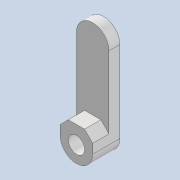
# Autodesk Inventor part: stand_1
Saved by Autodesk Inventor 2020 (Build 240168000, 168)
## iProperties
Created: 2021-07-20
Part Number: stand_1
Material: Generic
Document SubType Name: Modeling
Designer: Shuang Peng
Density: 1 g/cm^3
Appearance: Default
Author: Shuang Peng
Autodesk Inventor part; units mm, degrees
ref_plane "YZ Plane" through (0, 0, 0) normal (1, 0, 0) x (0, 1, 0)
ref_plane "XZ Plane" through (0, 0, 0) normal (0, 1, 0) x (-1, 0, 0)
ref_plane "XY Plane" through (0, 0, 0) normal (0, 0, 1) x (1, 0, 0)
sketch "Sketch1" plane through (0, 0, 0) normal (0, 0, 1) x (1, 0, 0)
  circle A0 centre (0, 0) radius 3
  line L0 (0, 0) -> (0, 30) construction
  line L1 (6, 0) -> (6, 30)
  line L2 (-6, 30) -> (-6, 0)
  arc A1 (-6, 0) -> (6, 0) centre (0, 0) ccw
  arc A2 (6, 30) -> (-6, 30) centre (0, 30) ccw
  point P0 (0, 15)
  dimension "d0" = 6
  dimension "d1" = 30
  dimension "d2" = 12
  constraints: 8 end point, 4 point on circle, 4 tangent, 3 centre point, 1 coincident, 1 midpoint, 1 parallel, 1 vertical
  measures "d0" diameter of A0
  measures "d1" distance of L0.start L0.end
  measures "d2" diameter of A2
extrude "Extrusion1" add sketch "Sketch1" along normal blind 10
sketch "Sketch2" plane through (0, 0, 10) normal (0, 0, 1) x (1, 0, 0)
  line L0 (-6, 30) -> (-6, 0) projected
  arc A0 (-6, 0) -> (6, 0) centre (0, 0) ccw projected
  line L1 (6, 0) -> (6, 30) projected
  arc A1 (6, 30) -> (-6, 30) centre (0, 30) ccw projected
  circle A2 centre (0, 0) radius 3 projected
  line L2 (13.5, 6.5) -> (13.5, -6.5)
  line L3 (13.5, -6.5) -> (-13.5, -6.5)
  line L4 (-13.5, -6.5) -> (-13.5, 6.5)
  line L5 (-13.5, 6.5) -> (13.5, 6.5)
  line L6 (13.5, 6.5) -> (-13.5, -6.5) construction
  line L7 (13.5, -6.5) -> (-13.5, 6.5) construction
  point P0 (-6, 6.5)
  point P1 (6, 6.5)
  dimension "d5" = 13
  dimension "d6" = 27
  constraints: 12 end point, 2 midpoint, 2 parallel, 1 perpendicular, 1 vertical
  measures "d5" distance of L2.start L2.end
  measures "d6" distance of L2.end L3.end
extrude "Extrusion2" cut sketch "Sketch2" against normal blind 6 contours A1 L1 L5 L0
chamfer "Chamfer1" distance 3 angle 45 2 edges at (-6, 6.5, 7) (6, 6.5, 7)
sketch "Sketch3" plane through (0, 0, 0) normal (0, 0, -1) x (-1, 0, 0)
  line L0 (6, 30) -> (6, 0) projected
  arc A0 (6, 30) -> (-6, 30) centre (0, 30) ccw projected
  line L1 (-6, 0) -> (-6, 30) projected
  arc A1 (-6, 0) -> (6, 0) centre (0, 0) ccw projected
  circle A2 centre (0, 0) radius 3 projected
  line L2 (6, 30) -> (6, 0) projected
  line L3 (-6, 30) -> (6, 30)
  constraints: 2 end point, 1 horizontal
extrude "Extrusion3" cut sketch "Sketch3" against normal blind 6 contours L3 A0
sketch "Sketch4" plane through (0, 0, 4) normal (0, 0, 1) x (1, 0, 0)
  line L0 (6, 30) -> (-6, 30) projected
  line L1 (-6, 3.5) -> (-6, 30) projected
  line L2 (-3, 6.5) -> (-6, 3.5) projected
  line L3 (3, 6.5) -> (-3, 6.5) projected
  line L4 (6, 3.5) -> (3, 6.5) projected
  line L5 (6, 30) -> (6, 3.5) projected
  arc A0 (-23.6294, 8.164) -> (-15.9746, 19.2305) centre (0, 0) ccw projected
  line L6 (6, 30) -> (6, 3.5) projected
  line L7 (6, 30) -> (18.1372, 17.2059)
  line L8 (-6, 30) -> (-18.1372, 17.2059)
  line L9 (4.0098, 35.0039) -> (10.8922, 27.749)
  line L10 (10.8922, 27.749) -> (7.9902, 24.9961)
  line L11 (7.9902, 24.9961) -> (1.1078, 32.251)
  line L12 (1.1078, 32.251) -> (4.0098, 35.0039)
  line L13 (6, 30) -> (-6, 30) projected
  line L14 (4.0098, 35.0039) -> (7.9902, 24.9961) construction
  line L15 (10.8922, 27.749) -> (1.1078, 32.251) construction
  line L16 (-1.1078, 32.251) -> (-7.9902, 24.9961)
  line L17 (-7.9902, 24.9961) -> (-10.8922, 27.749)
  line L18 (-10.8922, 27.749) -> (-4.0098, 35.0039)
  line L19 (-4.0098, 35.0039) -> (-1.1078, 32.251)
  line L20 (-1.1078, 32.251) -> (-10.8922, 27.749) construction
  line L21 (-7.9902, 24.9961) -> (-4.0098, 35.0039) construction
  line L22 (1.1078, 32.251) -> (-1.1078, 32.251)
  line L23 (6, 30) -> (2.5588, 33.6274)
  line L24 (-6, 30) -> (-2.5588, 33.6274)
  line L25 (7.9902, 24.9961) -> (-7.9902, 24.9961)
  point P0 (6, 24.9961)
  point P1 (9.4412, 26.3726)
  point P2 (-9.4412, 26.3726)
  point P3 (-6, 24.9961)
  point P4 (-6, 27.094)
  point P5 (-3.2432, 30)
  point P6 (3.2432, 30)
  point P7 (6, 27.094)
  dimension "d14" = 10
  dimension "d15" = 4
  dimension "d16" = 10
  dimension "d17" = 4
  constraints: 36 end point, 6 midpoint, 6 parallel, 3 perpendicular, 2 point on circle, 2 tangent
  measures "d14" distance of L9.start L9.end
  measures "d15" distance of L9.end L10.end
  measures "d16" distance of L16.start L16.end
  measures "d17" distance of L16.end L17.end
extrude "Extrusion4" add sketch "Sketch4" against normal blind 15 contours L5 L11 L0 | L7 L10 L11 L5 | L0 L11 L12 L23 | L0 L16 L22 L11 | L11 L25 L5 | L16 L1 L0 | L0 L24 L19 L16 | L1 L16 L17 L8 | L1 L25 L16
sketch "Sketch5" plane through (0, 0, -11) normal (0, 0, -1) x (-1, 0, 0)
  line L0 (1.1078, 32.251) -> (-1.1078, 32.251) projected
  line L1 (-1.1078, 32.251) -> (-2.5588, 33.6274) projected
  line L2 (-2.5588, 33.6274) -> (-9.4412, 26.3726) projected
  line L3 (-9.4412, 26.3726) -> (-7.9902, 24.9961) projected
  line L4 (-7.9902, 24.9961) -> (-6, 24.9961) projected
  line L5 (-6, 24.9961) -> (-6, 27.094) projected
  line L6 (-6, 27.094) -> (-3.2432, 30) projected
  line L7 (-3.2432, 30) -> (3.2432, 30) projected
  line L8 (3.2432, 30) -> (6, 27.094) projected
  line L9 (6, 27.094) -> (6, 24.9961) projected
  line L10 (6, 24.9961) -> (7.9902, 24.9961) projected
  line L11 (7.9902, 24.9961) -> (9.4412, 26.3726) projected
  line L12 (9.4412, 26.3726) -> (2.5588, 33.6274) projected
  line L13 (2.5588, 33.6274) -> (1.1078, 32.251) projected
  line L14 (-7.9902, 24.9961) -> (-6, 27.094)
  line L15 (7.9902, 24.9961) -> (6, 27.094)
  point P0 (0, 0)
  constraints: 4 end point
extrude "Extrusion5" cut sketch "Sketch5" against normal up to surface (11 mm away) contours L10 L9 L15 | L14 L5 L4
thicken "Thicken1" operation add thickness 1 both sides no extend neighbours yes toward (0.6882359, 0.7254869, 0) faces at (-8.9575, 25.9137, -2.3333)
thicken "Thicken2" operation add thickness 1 both sides no extend neighbours yes toward (-0.6882359, 0.7254869, 0) faces at (8.9575, 25.9137, -2.3333)
sketch "Sketch6" plane through (-1.1078, 32.251, 4) normal (0.6882359, 0.7254869, 0) x (0.7254869, -0.6882359, 0)
  line L0 (-2, 12.5) -> (-3.1464, 13.6464)
  line L1 (-3.1464, 11.3536) -> (-2, 12.5)
  line L2 (-2, 0) -> (-2, 15) projected
  circle A0 centre (-2, 12.5) radius 1.25
  point P0 (23, 4)
  point P1 (-2, 13.75)
  point P2 (-2, 11.25)
  dimension "d27" = 2.5
  constraints: 4 end point, 1 centre point, 1 coincident, 5 other
  measures "d27" diameter of A0
extrude "Extrusion6" cut sketch "Sketch6" against normal blind 15 contours L2 A0
sketch "Sketch7" plane through (-1.1078, 32.251, 4) normal (0.6882359, 0.7254869, 0) x (0.7254869, -0.6882359, 0)
  line L0 (-2, 8.5) -> (-3.1464, 7.3536)
  line L1 (-3.1464, 9.6464) -> (-2, 8.5)
  line L2 (-2, 0) -> (-2, 11.25) projected
  circle A0 centre (-2, 8.5) radius 1.25
  point P0 (23, 4)
  point P1 (-2, 9.75)
  point P2 (-2, 7.25)
  dimension "d30" = 2.5
  constraints: 4 end point, 1 centre point, 1 coincident, 5 other
  measures "d30" diameter of A0
extrude "Extrusion7" cut sketch "Sketch7" against normal blind 15 contours L2 A0
chamfer "Chamfer2" distance 2 angle 45 2 edges at (-5.6559, 30.3627, 4) (5.6559, 30.3627, 4)
sketch "Sketch8" plane through (0, 0, -11) normal (0, 0, -1) x (-1, 0, 0)
  arc A0 (23.3037, 11.8564) -> (25.9335, 3.3299) centre (0, 0) ccw projected
  circle A1 centre (0, 0) radius 3 projected
  line L0 (7.302, 25.7216) -> (3.2432, 30) projected
  line L1 (3.2432, 30) -> (-3.2432, 30) projected
  line L2 (-3.2432, 30) -> (-7.302, 25.7216) projected
  line L3 (-7.302, 25.7216) -> (-6.5372, 24.9961) projected
  line L4 (-6, 24.9961) -> (-6.5372, 24.9961) projected
  line L5 (-6, 0) -> (-6, 24.9961) projected
  arc A2 (-6, 0) -> (6, 0) centre (0, 0) ccw projected
  line L6 (6, 24.9961) -> (6, 0) projected
  line L7 (6.5372, 24.9961) -> (6, 24.9961) projected
  line L8 (6.5372, 24.9961) -> (7.302, 25.7216) projected
  line L9 (-5.2726, 27.8608) -> (5.2726, 27.8608)
  constraints: 2 end point, 2 midpoint
extrude "Extrusion8" add sketch "Sketch8" against normal up to surface (11 mm away) contours L9 L2 L1 L0
ref_plane "Work Plane2" through (0, 36.3248, -3.25) normal (-1, 0, 0) x (0, 0, 1)
mirror "Mirror2" about plane through (0, 36.3248, -3.25) normal (-1, 0, 0) of "Extrusion7", "Extrusion6"
thicken "Thicken3" operation add thickness 1 both sides no extend neighbours yes toward (0, 1, 0) faces at (1.7575, 27.8608, -7.3333)
thicken "Thicken4" operation add thickness 2 both sides no extend neighbours yes toward (0, 0, -1) faces at (0.3693, 29.9908, -11)
fillet "Fillet2" radius 3 2 edges at (-6, 24.9961, 2) (6, 24.9961, 2)
fillet "Fillet3" radius 3 3 edges at (-5.813, 27.2912, 0) (0, 28.8608, 0) (5.813, 27.2912, 0)
sketch "Sketch9" plane through (-2.5588, 33.6274, -13) normal (-0.7254869, 0.6882359, 0) x (0, 0, 1)
  line L0 (3.25, -9) -> (3.25, 0) projected
  line L1 (3.25, 0) -> (0, 0) projected
  line L2 (0, -9) -> (0, 0) projected
  line L3 (3.25, -9) -> (0, -9) projected
  line L4 (15, 0) -> (15, -9) projected
  line L5 (15, 0) -> (9.75, 0) projected
  line L6 (9.75, 0) -> (9.75, -9) projected
  line L7 (15, -9) -> (9.75, -9) projected
  line L8 (3.25, -9) -> (3.25, 0) projected
  line L9 (17, 0) -> (0, 0) projected
  line L10 (3.25, 0) -> (0, 0)
  line L11 (1.625, 0) -> (1.625, -9)
  line L12 (10, -9) -> (0, -9) projected
  line L13 (1.625, -3) -> (1.625, -6) construction
  line L14 (1.275, -3) -> (1.275, -6)
  line L15 (1.975, -6) -> (1.975, -3)
  arc A0 (1.975, -3) -> (1.275, -3) centre (1.625, -3) ccw
  arc A1 (1.275, -6) -> (1.975, -6) centre (1.625, -6) ccw
  line L16 (1.625, -4.5) -> (11.125, -4.5)
  line L17 (11.125, -3) -> (11.125, -6) construction
  line L18 (10.775, -3) -> (10.775, -6)
  line L19 (11.475, -6) -> (11.475, -3)
  arc A2 (11.475, -3) -> (10.775, -3) centre (11.125, -3) ccw
  arc A3 (10.775, -6) -> (11.475, -6) centre (11.125, -6) ccw
  point P0 (13, -22.6352)
  dimension "d44" = 1.5
  dimension "d45" = 0.7
  dimension "d46" = 9.5
  dimension "d47" = 1.5
  dimension "d48" = 0.7
  constraints: 22 end point, 8 point on circle, 8 tangent, 4 centre point, 4 midpoint, 2 parallel, 2 perpendicular, 2 point on line, 1 horizontal, 1 vertical
  measures "d44" distance of L16.start L13.end
  measures "d45" diameter of A1
  measures "d46" distance of L16.start L16.end
  measures "d47" distance of L16.end L17.end
  measures "d48" diameter of A3
extrude "Extrusion9" cut sketch "Sketch9" against normal blind 15 contours L16 L11 A0 L15 | L15 A1 L11 L16 | A1 L14 A0 L11 | A2 L19 A3 L18
mirror "Mirror3" about plane through (0, 36.3248, -3.25) normal (-1, 0, 0) of "Extrusion9"
fillet "Fillet4" radius 2 8 edges at (4.3239, 28.8608, -12.3625) (4.313, 28.8352, -2.6092) (4.3239, 28.8608, -7.0125) (3.6847, 27.3732, -0.4092) (-3.6847, 27.3732, -0.4092) (-4.313, 28.8352, -2.6092) (-4.3239, 28.8608, -7.0125) (-4.3239, 28.8608, -12.3625)
ref_plane "Work Plane3" through (0, 0, 8) normal (0, 0, 1) x (1, 0, 0)
sketch "Sketch10" plane through (0, 0, 8) normal (0, 0, 1) x (1, 0, 0)
  circle A0 centre (0, 0) radius 3 projected
  circle A1 centre (0, 0) radius 2
  dimension "d53" = 1
  constraints: 1 centre point, 1 coincident
  measures "d53" radial gap between concentric circles of A0 A1
extrude "Extrusion10" add sketch "Sketch10" against normal blind 6
chamfer "Chamfer3" distance 1 angle 45 2 edges at (-2, 0, 8) (-2, 0, 2)
thicken "Thicken5" operation add thickness 1 both sides no extend neighbours yes toward (0, -1, 0) faces at (-1, 6.5, 8)
sketch "Sketch11" plane through (0, 0, 4) normal (0, 0, 1) x (1, 0, 0)
  line L0 (1.1078, 32.251) -> (7.302, 25.7216) projected
  line L1 (1.1078, 32.251) -> (-1.1078, 32.251) projected
  line L2 (-7.302, 25.7216) -> (-1.1078, 32.251) projected
  line L3 (-7.302, 25.7216) -> (-6.5372, 24.9961) projected
  arc A0 (-6, 23.283) -> (-6.5372, 24.9961) centre (-9, 23.283) ccw projected
  line L4 (-6, 3.5) -> (-6, 23.283) projected
  line L5 (-4, 5.5) -> (-6, 3.5) projected
  line L6 (4, 5.5) -> (-4, 5.5) projected
  line L7 (6, 3.5) -> (4, 5.5) projected
  line L8 (6, 23.283) -> (6, 3.5) projected
  arc A1 (6.5372, 24.9961) -> (6, 23.283) centre (9, 23.283) ccw projected
  line L9 (6.5372, 24.9961) -> (7.302, 25.7216) projected
  line L10 (0, 32.251) -> (0, 27.251)
  line L11 (0, 27.251) -> (0, 21.251)
  line L12 (0, 21.251) -> (0, 9.251)
  circle A2 centre (0, 27.251) radius 1.5
  circle A3 centre (0, 21.251) radius 1.5
  circle A4 centre (0, 9.251) radius 1.5
  line L13 (0, 15.251) -> (3, 15.251)
  circle A5 centre (3, 15.251) radius 1.5
  line L14 (0, 15.251) -> (-3, 15.251)
  circle A6 centre (-3, 15.251) radius 1.5
  point P0 (0, 0)
  dimension "d61" = 5
  dimension "d62" = 6
  dimension "d63" = 12
  dimension "d64" = 3
  dimension "d65" = 3
  dimension "d66" = 3
  dimension "d67" = 3
  dimension "d68" = 3
  dimension "d69" = 3
  dimension "d70" = 3
  constraints: 10 end point, 5 centre point, 5 coincident, 2 horizontal, 2 midpoint, 2 point on line, 1 vertical
  measures "d61" distance of L10.start L10.end
  measures "d62" distance of L10.end L11.end
  measures "d63" distance of L11.end L12.end
  measures "d64" diameter of A2
  measures "d65" diameter of A3
  measures "d66" diameter of A4
  measures "d67" distance of L13.start L13.end
  measures "d68" diameter of A5
  measures "d69" distance of L13.start L14.end
  measures "d70" diameter of A6
extrude "Extrusion11" cut sketch "Sketch11" against normal blind 6 contours A3 L12 L11 | L11 L12 A3 | A4 | A5 | A6
fillet "Fillet5" radius 1 3 edges at (5, 4.5, 4) (0, 5.5, 4) (-5, 4.5, 4)
chamfer "Chamfer4" distance 0.5 angle 45 2 edges at (-3, 0, 10) (-3, 0, 0)
body "Solid1"
